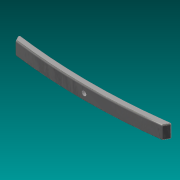
# Autodesk Inventor part: LEAF 6
Saved by Autodesk Inventor 2014 SP2 (Build 180246200, 246)
## iProperties
Created: 2019-07-17
Part Number: LEAF 6
Material: Steel, Carbon
Document SubType Name: Modeling
Designer: USER PC
Density: 7.87 g/cm^3
Appearance: Semi-Polished
Author: USER PC
Autodesk Inventor part; units mm, degrees
ref_plane "YZ Plane" through (0, 0, 0) normal (1, 0, 0) x (0, 1, 0)
ref_plane "XZ Plane" through (0, 0, 0) normal (0, 1, 0) x (-1, 0, 0)
ref_plane "XY Plane" through (0, 0, 0) normal (0, 0, 1) x (1, 0, 0)
sketch "Sketch1" plane through (0, 0, 0) normal (0, 0, 1) x (1, 0, 0)
  arc A0 (0.1634, -151.6592) -> (162.48, -141.1714) centre (0.1634, 1109.6463) ccw
  arc A1 (0.1634, -136.6592) -> (171.9535, -124.7627) centre (0.1634, 1109.6463) ccw
  line L0 (171.9535, -124.7627) -> (162.48, -141.1714)
  line L1 (171.9535, -124.7627) -> (190.9007, -124.7627) construction
  line L2 (0.1634, -151.6592) -> (0.1634, -124.7627)
  arc A2 (-162.1531, -141.1714) -> (0.1634, -151.6592) centre (0.1634, 1109.6463) ccw
  arc A3 (-171.6266, -124.7627) -> (0.1634, -136.6592) centre (0.1634, 1109.6463) ccw
  line L3 (-171.6266, -124.7627) -> (-162.1531, -141.1714)
  point P0 (0, 0)
  dimension "d0" = 15
  dimension "d1" = 120
  constraints: 8 end point, 8 point on circle, 4 centre point, 2 symmetric about line, 1 equal length, 1 horizontal, 1 perpendicular, 2 other
  measures "d0" radial gap between concentric circles of A0 A1
  measures "d1" angle of L0 L1
extrude "Extrusion1" add sketch "Sketch1" along normal blind 30
fillet "Fillet1" radius 3 12 edges at (-85.9373, -133.6816, 30) (81.4909, -149.0346, 30) (167.2167, -132.9671, 30) (171.9535, -124.7627, 15) (162.48, -141.1714, 15) (167.2167, -132.9671, 0) (-166.8899, -132.9671, 30) (-171.6266, -124.7627, 15) (86.2642, -133.6816, 0) (81.4909, -149.0346, 0) (-162.1531, -141.1714, 15) (-166.8899, -132.9671, 0)
sketch "Sketch2" plane through (0, 0, 0) normal (0, 1, 0) x (-1, 0, 0)
  line L0 (0, 0) -> (0, 15)
  circle A0 centre (0, 15) radius 5
  dimension "d5" = 15
  dimension "d6" = 10
  constraints: 2 end point, 1 centre point, 1 coincident, 1 vertical
  measures "d5" distance of L0.start L0.end
  measures "d6" diameter of A0
extrude "Extrusion2" cut sketch "Sketch2" against normal blind 300
body "Solid1"
